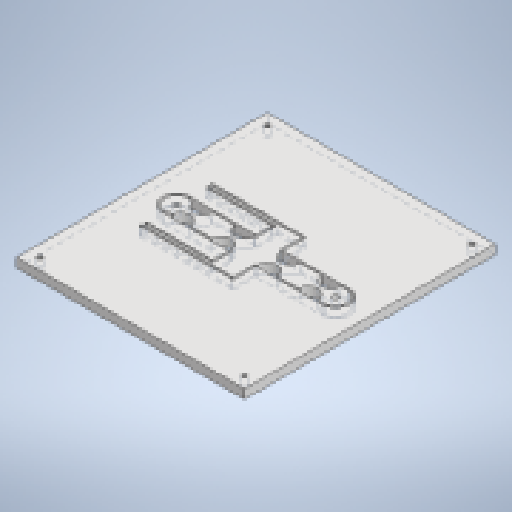
# Autodesk Inventor part: FlexK7Holder
Saved by Autodesk Inventor 2023 (Build 270158000, 158)
## iProperties
Created: 2023-03-30
Part Number: FlexK7Holder
Material: Generic
Document SubType Name: Modeling
Designer: Nathann
Density: 1 g/cm^3
Appearance: Default
Author: Nathann
Autodesk Inventor part; units mm, degrees
ref_plane "YZ Plane" through (0, 0, 0) normal (1, 0, 0) x (0, 1, 0)
ref_plane "XZ Plane" through (0, 0, 0) normal (0, 1, 0) x (-1, 0, 0)
ref_plane "XY Plane" through (0, 0, 0) normal (0, 0, 1) x (1, 0, 0)
sketch "Sketch1" plane through (0, 0, 0) normal (0, 1, 0) x (-1, 0, 0)
  line L0 (0, 0) -> (-100, 0)
  line L1 (-100, 0) -> (-100, -110)
  line L2 (-100, -110) -> (0, -110)
  line L3 (0, -110) -> (0, 0)
  dimension "d0" = 110
  dimension "d1" = 100
  constraints: 8 end point, 2 parallel, 1 horizontal, 1 perpendicular
  measures "d0" distance of L0.end L1.end
  measures "d1" distance of L0.start L0.end
extrude "Extrusion1" add sketch "Sketch1" along normal blind 4
sketch "Sketch5" plane through (0, 4, 0) normal (0, 1, 0) x (1, 0, 0)
  circle A0 centre (5, 5) radius 1.1
  line L0 (0, 0) -> (100, 0) projected
  line L1 (0, 110) -> (0, 0) projected
  line L2 (0, 55) -> (10.2566, 55)
  circle A1 centre (5, 105) radius 1.1
  line L3 (0, 110) -> (100, 110)
  line L4 (0, 0) -> (0, 110)
  line L5 (50, 0) -> (50, 7.5266)
  circle A2 centre (95, 5) radius 1.1
  line L6 (100, 110) -> (100, 0)
  circle A3 centre (95, 105) radius 1.1
  line L7 (100, 0) -> (100, 110)
  point P0 (100, 55)
  point P1 (89.7434, 55)
  dimension "d41" = 5
  dimension "d42" = 5
  dimension "d43" = 2.2
  constraints: 12 end point, 12 symmetric about line, 4 centre point, 2 midpoint, 1 horizontal, 1 vertical, 3 other
  measures "d41" distance from line of L0 A0.centre
  measures "d42" distance from line of A0.centre L1
  measures "d43" diameter of A0
extrude "Extrusion4" cut sketch "Sketch5" against normal blind 10 contours A0 | A1 | A2 | A3
thread "Thread7" size "M2.5x0.45" class "6H" standard "ANSI Metric M Profile" length 10
thread "Thread8" size "M2.5x0.45" class "6H" standard "ANSI Metric M Profile" length 10
thread "Thread9" size "M2.5x0.45" class "6H" standard "ANSI Metric M Profile" length 10
thread "Thread10" size "M2.5x0.45" class "6H" standard "ANSI Metric M Profile" length 10
sketch "Sketch6" plane through (0, 0, 0) normal (0, -1, 0) x (1, 0, 0)
  line L0 (0, 0) -> (100, 0) projected
  line L1 (0, -110) -> (0, 0) projected
  line L2 (47.5, -85) -> (52.5, -85)
  line L3 (52.5, -85) -> (52.5, -25)
  line L4 (52.5, -25) -> (47.5, -25)
  line L5 (47.5, -25) -> (47.5, -85)
  line L6 (47.5, -85) -> (52.5, -25) construction
  line L7 (52.5, -85) -> (47.5, -25) construction
  line L8 (100, 0) -> (100, -110) projected
  line L9 (100, -110) -> (0, -110) projected
  line L10 (47.5, -25) -> (7.5, -25)
  line L11 (7.5, -25) -> (7.5, -26)
  line L12 (7.5, -26) -> (47.5, -26)
  line L13 (47.5, -26) -> (47.5, -25)
  line L14 (47.5, -85) -> (7.5, -85)
  line L15 (7.5, -85) -> (7.5, -84)
  line L16 (7.5, -84) -> (47.5, -84)
  line L17 (47.5, -84) -> (47.5, -85)
  line L18 (47.5, -28) -> (20, -28)
  line L19 (20, -28) -> (20, -33)
  line L20 (20, -33) -> (47.5, -33)
  line L21 (47.5, -33) -> (47.5, -28)
  line L22 (52.5, -28) -> (80, -28)
  line L23 (80, -28) -> (80, -33)
  line L24 (80, -33) -> (52.5, -33)
  line L25 (52.5, -33) -> (52.5, -28)
  line L26 (65.25, -52.5) -> (80, -52.5)
  line L27 (80, -52.5) -> (80, -57.5)
  line L28 (80, -57.5) -> (65.25, -57.5)
  line L29 (65.25, -57.5) -> (65.25, -52.5)
  line L30 (20, -57.5) -> (34.75, -57.5)
  line L31 (34.75, -57.5) -> (34.75, -52.5)
  line L32 (34.75, -52.5) -> (20, -52.5)
  line L33 (20, -52.5) -> (20, -57.5)
  line L34 (20, -52.5) -> (21, -52.5)
  line L35 (21, -52.5) -> (21, -33)
  line L36 (21, -33) -> (20, -33)
  line L37 (20, -33) -> (20, -52.5)
  line L38 (34.75, -52.5) -> (33.75, -52.5)
  line L39 (33.75, -52.5) -> (33.75, -33)
  line L40 (33.75, -33) -> (34.75, -33)
  line L41 (34.75, -33) -> (34.75, -52.5)
  line L42 (65.25, -52.5) -> (66.25, -52.5)
  line L43 (66.25, -52.5) -> (66.25, -33)
  line L44 (66.25, -33) -> (65.25, -33)
  line L45 (65.25, -33) -> (65.25, -52.5)
  line L46 (80, -33) -> (79, -33)
  line L47 (79, -33) -> (79, -52.5)
  line L48 (79, -52.5) -> (80, -52.5)
  line L49 (80, -52.5) -> (80, -33)
  line L50 (80, -52.5) -> (85, -52.5)
  line L51 (85, -52.5) -> (85, -57.5)
  line L52 (85, -57.5) -> (80, -57.5)
  line L53 (80, -57.5) -> (80, -52.5)
  arc A0 (85, -57.5) -> (85, -52.5) centre (85, -55) ccw
  line L54 (20, -57.5) -> (15, -57.5)
  line L55 (15, -57.5) -> (15, -52.5)
  line L56 (15, -52.5) -> (20, -52.5)
  line L57 (20, -52.5) -> (20, -57.5)
  arc A1 (15, -52.5) -> (15, -57.5) centre (15, -55) ccw
  circle A2 centre (85, -55) radius 1.1
  circle A3 centre (15, -55) radius 1.1
  line L58 (7.5, -26) -> (7.5, -84)
  line L59 (52.5, -28) -> (92.5, -28)
  line L60 (92.5, -28) -> (92.5, -85)
  line L61 (92.5, -85) -> (52.5, -85)
  line L62 (52.5, -85) -> (52.5, -28)
  line L63 (7.5, -25) -> (92.5, -25)
  line L64 (92.5, -25) -> (92.5, -24)
  line L65 (92.5, -24) -> (7.5, -24)
  line L66 (7.5, -24) -> (7.5, -25)
  line L67 (7.5, -85) -> (92.5, -85)
  line L68 (92.5, -85) -> (92.5, -86)
  line L69 (92.5, -86) -> (7.5, -86)
  line L70 (7.5, -86) -> (7.5, -85)
  line L71 (92.5, -28) -> (92.5, -25)
  circle A4 centre (82, -52.5) radius 2
  circle A5 centre (82, -57.5) radius 2
  circle A6 centre (18, -52.5) radius 2
  circle A7 centre (18, -57.5) radius 2
  line L72 (47.5, -60.5) -> (7.5, -60.5)
  line L73 (7.5, -60.5) -> (7.5, -59.5)
  line L74 (7.5, -59.5) -> (47.5, -59.5)
  line L75 (47.5, -59.5) -> (47.5, -60.5)
  point P0 (50, -55)
  point P1 (72.625, -52.5)
  point P2 (65.25, -55)
  point P3 (16, -52.5)
  point P4 (16, -57.5)
  point P5 (84, -57.5)
  point P6 (84, -52.5)
  point P7 (47.5, -59.5)
  dimension "d113" = 50
  dimension "d114" = 55
  dimension "d115" = 5
  dimension "d116" = 60
  dimension "d117" = 1
  dimension "d118" = 2
  dimension "d119" = 40
  dimension "d120" = 27.5
  dimension "d121" = 40
  dimension "d122" = 1
  dimension "d123" = 5
  dimension "d124" = 0
  dimension "d125" = 5
  dimension "d126" = 27.5
  dimension "d127" = 1
  dimension "d128" = 1
  dimension "d129" = 1
  dimension "d130" = 1
  dimension "d131" = 5
  dimension "d132" = 5
  dimension "d133" = 0
  dimension "d134" = 19.5
  dimension "d135" = 70
  dimension "d136" = 5
  dimension "d138" = 5
  dimension "d139" = 2.2
  dimension "d140" = 2.2
  dimension "d141" = 40
  dimension "d142" = 1
  dimension "d143" = 1
  dimension "d144" = 4
  dimension "d145" = 4
  dimension "d146" = 3
  dimension "d147" = 3
  dimension "d148" = 3
  dimension "d149" = 4
  dimension "d150" = 4
  dimension "d151" = 1
  dimension "d152" = 2
  constraints: 144 end point, 34 parallel, 17 horizontal, 17 perpendicular, 14 point on line, 8 centre point, 8 midpoint, 4 point on circle, 2 coincident, 2 vertical, 1 vertical alignment
  measures "d113" distance from line of L8 point (50, -55)
  measures "d114" distance from line of L9 point (50, -55)
  measures "d115" distance of L3.end L4.end
  measures "d116" distance of L2.end L3.end
  measures "d117" distance between parallel lines of L10 L12
  measures "d118" distance between parallel lines of L12 L18
  measures "d119" distance of L4.end L10.end
  measures "d120" distance of L19.end L20.end
  measures "d121" distance of L2.start L14.end
  measures "d122" distance between parallel lines of L14 L16
  measures "d123" distance between parallel lines of L20 L18
  measures "d124" distance between parallel lines of L18 L22
  measures "d125" distance between parallel lines of L22 L24
  measures "d126" distance of L22.start L22.end
  measures "d127" distance between parallel lines of L39 L41
  measures "d128" distance between parallel lines of L49 L47
  measures "d129" distance between parallel lines of L45 L43
  measures "d130" distance between parallel lines of L37 L35
  measures "d131" distance from line of L28 point (72.625, -52.5)
  measures "d132" distance between parallel lines of L30 L32
  measures "d133" vertical distance of point (50, -55) point (65.25, -55)
  measures "d134" distance between parallel lines of L24 L26
  measures "d135" distance of A1.centre A0.centre
  measures "d136" distance from line of L27 A0.centre
  measures "d138" distance from line of A1.centre L33
  measures "d139" diameter of A2
  measures "d140" diameter of A3
  measures "d141" distance between parallel lines of L62 L60
  measures "d142" distance between parallel lines of L67 L69
  measures "d143" distance between parallel lines of L65 L63
  measures "d144" diameter of A4
  measures "d145" diameter of A5
  measures "d146" horizontal distance of A0.centre A4.centre
  measures "d147" horizontal distance of A6.centre A1.centre
  measures "d148" horizontal distance of A1.centre A7.centre
  measures "d149" diameter of A7
  measures "d150" diameter of A6
  measures "d151" distance between parallel lines of L72 L74
  measures "d152" distance between parallel lines of L30 L74
extrude "Extrusion5" cut sketch "Sketch6" against normal blind 4 contours L2 L61 L68 L69 L70 L14 | L3 L24 L45 L29 L28 A5 L52 A0 L50 A4 L49 L23 L59 L60 L61 | L16 L58 L72 L5 | L3 L63 L71 L59 L22 | L74 A7 L30 L31 L41 L20 L5 | L4 L10 L66 L65 L64 L63 | L24 L47 L26 L43 | L74 L58 L12 L5 L18 L19 L37 A6 L56 A1 L54 A7 | A7 L54 | A7 L54 | A4 L50 | L50 A4 | A5 L52 | L52 A5 | L39 L32 L35 L20 | A6 L56 | L56 A6 | A3 L55 | L55 A3 | A2 L51 | L51 A2
sketch "Sketch8" plane through (0, 4, 0) normal (0, 1, 0) x (1, 0, 0)
  line L0 (100, 110) -> (0, 110) projected
  line L1 (60.5042, 110) -> (30.5042, 110)
  line L2 (30.5042, 110) -> (30.5042, 96.3922)
  line L3 (30.5042, 96.3922) -> (60.5042, 96.3922)
  line L4 (60.5042, 96.3922) -> (60.5042, 110)
  line L5 (0, 110) -> (0, 0) projected
  line L6 (60.5042, 96.3922) -> (0, 96.3922)
  line L7 (0, 96.3922) -> (0, 91.3922)
  line L8 (0, 91.3922) -> (60.5042, 91.3922)
  line L9 (60.5042, 91.3922) -> (60.5042, 96.3922)
  line L10 (0, 91.3922) -> (5, 91.3922)
  line L11 (5, 91.3922) -> (5, 31)
  line L12 (5, 31) -> (0, 31)
  line L13 (0, 31) -> (0, 91.3922)
  line L14 (7.5, 60.5) -> (7.5, 84) projected
  line L15 (5, 31) -> (7.5, 31)
  line L16 (7.5, 31) -> (7.5, 79)
  line L17 (7.5, 79) -> (5, 79)
  line L18 (5, 79) -> (5, 31)
  line L19 (7.5, 84) -> (47.5, 84) projected
  line L20 (47.5, 26) -> (7.5, 26) projected
  line L21 (7.5, 80) -> (6, 80)
  line L22 (6, 80) -> (6, 90.3922)
  line L23 (6, 90.3922) -> (61.5042, 90.3922)
  line L24 (61.5042, 90.3922) -> (61.5042, 110)
  line L25 (0, 97.2327) -> (28.374, 97.2327)
  line L26 (28.374, 97.2327) -> (28.374, 110)
  line L27 (7.5, 26) -> (7.5, 59.5) projected
  line L28 (7.5, 30) -> (0, 30)
  point P0 (6.25, 79)
  point P1 (0, 31)
  point P2 (0, 96.3922)
  point P3 (5, 91.3922)
  dimension "d153" = 5
  dimension "d154" = 5
  dimension "d155" = 5
  dimension "d156" = 5
  dimension "d157" = 30
  dimension "d158" = 1
  dimension "d159" = 1
  dimension "d160" = 1
  dimension "d161" = 1
  dimension "d162" = 1
  constraints: 46 end point, 9 parallel, 9 point on line, 8 perpendicular, 6 horizontal, 1 midpoint
  measures "d153" distance between parallel lines of L19 L17
  measures "d154" distance between parallel lines of L15 L20
  measures "d155" distance between parallel lines of L5 L11
  measures "d156" distance between parallel lines of L8 L6
  measures "d157" distance between parallel lines of L2 L4
  measures "d158" distance from line of L28 L11.end
  measures "d159" distance from line of point (6.25, 79) L21
  measures "d160" distance between parallel lines of L11 L22
  measures "d161" distance between parallel lines of L23 L8
  measures "d162" distance between parallel lines of L24 L4
extrude "Extrusion6" cut sketch "Sketch8" against normal blind 4 contours L24 L23 L22 L21 L14 L17 L11 L8 L9 L4 L0 | L2 L6 L5 L25 L26 L0 | L12 L15 L27 L28 L5
body "Solid1"
